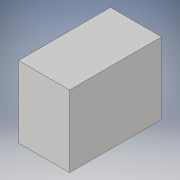
# Autodesk Inventor part: Electronics_Box
Saved by Autodesk Inventor 2018 (Build 220112000, 112)
## iProperties
Created: 2019-07-25
Part Number: Electronics_Box
Material: Generic
Document SubType Name: Modeling
Designer: micha
Density: 1 g/cm^3
Appearance: Default
Author: micha
Autodesk Inventor part; units mm, degrees
ref_plane "YZ Plane" through (0, 0, 0) normal (1, 0, 0) x (0, 1, 0)
ref_plane "XZ Plane" through (0, 0, 0) normal (0, 1, 0) x (-1, 0, 0)
ref_plane "XY Plane" through (0, 0, 0) normal (0, 0, 1) x (1, 0, 0)
sketch "Sketch1" plane through (0, 0, 0) normal (0, 1, 0) x (-1, 0, 0)
  line L0 (0, 0) -> (127, 0)
  line L1 (127, 0) -> (127, -228.6)
  line L2 (127, -228.6) -> (0, -228.6)
  line L3 (0, -228.6) -> (0, 0)
  dimension "d0" = 127
  dimension "d1" = 228.6
  constraints: 8 end point, 2 parallel, 1 horizontal, 1 perpendicular
  measures "d0" distance of L1.end L2.end
  measures "d1" distance of L0.end L1.end
extrude "Extrusion1" add sketch "Sketch1" along normal blind 177.8
sketch "Sketch2" plane through (0, 0, -228.6) normal (0, 0, -1) x (-1, 0, 0)
  line L0 (127, 0) -> (0, 0) projected
  line L1 (127, 0) -> (127, 177.8) projected
  line L2 (0, 177.8) -> (127, 177.8) projected
  line L3 (0, 0) -> (0, 177.8) projected
  line L4 (114.3, 165.1) -> (114.3, 12.7)
  line L5 (114.3, 12.7) -> (12.7, 12.7)
  line L6 (12.7, 12.7) -> (12.7, 165.1)
  line L7 (12.7, 165.1) -> (114.3, 165.1)
  dimension "d4" = 12.7
  constraints: 8 end point, 3 other
  measures "d4" distance between parallel lines of L2 L7
shell "Shell1" thickness 3.175 removed faces 1 at (-84.6667, 59.2667, -228.6)
extrude "Extrusion2" add sketch "Sketch2" against normal blind 3.175
body "Solid1"
